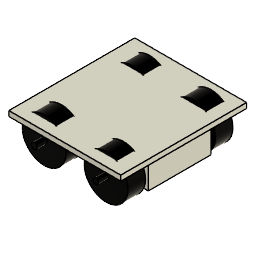
Bottom (Autodesk Fusion 360 design; units mm, degrees)
part number: 2026-06-28-07-39-42-404
Autodesk Fusion 360 part; units mm, degrees
sketch "Sketch1" plane through (0, 0, 0) normal (0, 0, 1) x (1, 0, 0)
  line L0 (0, 0) -> (72, 0)
  line L1 (72, 0) -> (72, 64)
  line L2 (72, 64) -> (0, 64)
  line L3 (0, 64) -> (0, 0)
  point P0 (9, 50)
  point P1 (63, 50)
  point P2 (9, 14)
  point P3 (63, 14)
  dimension "d1" = 72
  dimension "d2" = 64
  constraint horizontal L0
  constraint vertical L1
  constraint horizontal L2
  constraint vertical L3
  constraint coincident L0.start L3.end
  measures "d1" distance of L0.start L0.end
  measures "d2" distance of L0.start L2.end
extrude "Extrude1" add sketch "Sketch1" along normal blind 3 makes body 1
sketch "Sketch2" plane through (0, 0, 3) normal (0, 0, 1) x (-1, 0, 0)
  line L0 (0, -64) -> (0, 0)
  line L1 (0, 0) -> (-72, 0)
  line L2 (-72, 0) -> (-72, -64)
  line L3 (-72, -64) -> (0, -64)
  point P0 (-9, -50)
  point P1 (-9, -14)
  point P2 (-63, -49.8902)
  point P3 (-63, -14)
hole "Hole1" at (9, 50, 3) at (63, 49.8902, 3) at (63, 14, 3) at (9, 14, 3) direction (0, 0, -1) diameter 3.4 depth 3 tip angle 180 bodies 1
sketch "Sketch3" plane through (0, 0, 0) normal (0, 0, 1) x (1, 0, 0)
sketch "Sketch4" plane through (0, 0, 0) normal (1, 0, 0) x (0, 1, 0)
  line L0 (0, 11.5) -> (-48, 11.5)
  arc A0 (-48, 11.5) -> (-48, -11.5) centre (-48, 0) ccw
  line L1 (-48, -11.5) -> (0, -11.5)
  arc A1 (0, -11.5) -> (0, 11.5) centre (0, 0) ccw
  line L2 (0, 0) -> (-48, 0) construction
  dimension "d21" = 23
  constraint tangent L0 A0
  constraint tangent A0 L1
  constraint parallel L0 L1
  constraint tangent L1 A1
  constraint tangent L0 A1
  constraint horizontal L2
  constraint coincident A1.centre L2.start
  measures "d21" diameter of A0
ref_plane "WorkPlane1" through (0, -21.8422, 11.5) normal (0, -1, 0) x (1, 0, 0)
sketch "Sketch5" plane through (0, -21.8422, 11.5) normal (0, -1, 0) x (1, 0, 0)
  line L0 (0, 0) -> (-20, 0)
  line L1 (-20, 0) -> (-20, -2)
  line L2 (-20, -2) -> (0, -2)
  line L3 (0, -2) -> (0, 0)
  dimension "d23" = 2
  constraint horizontal L0
  constraint vertical L1
  constraint horizontal L2
  constraint vertical L3
  constraint coincident L0.start L3.end
  measures "d23" distance of L0.start L2.end
sketch "Sketch6" plane through (0, 0, 31.5) normal (0, 0, 1) x (-1, 0, 0)
sketch "Sketch7" plane through (0, 0, 31.5) normal (0, 0, 1) x (-1, 0, 0)
  line L0 (14.9741, -0.5329) -> (34.9741, -0.5329)
  line L1 (34.9741, -0.5329) -> (34.9741, 8.4671)
  line L2 (34.9741, 8.4671) -> (14.9741, 8.4671)
  line L3 (14.9741, 8.4671) -> (14.9741, -0.5329)
  dimension "d30" = 20
  dimension "d31" = 9
  constraint horizontal L0
  constraint vertical L1
  constraint horizontal L2
  constraint vertical L3
  measures "d30" distance of L0.start L0.end
  measures "d31" distance of L0.start L2.end
sketch "Sketch8" plane through (0, 0, 0) normal (1, 0, 0) x (0, 1, 0)
  circle A0 centre (-10, -10) radius 11
  dimension "d36" = 22
  measures "d36" diameter of A0
sketch "Sketch9" plane through (0, 0, 0) normal (1, 0, 0) x (0, 1, 0)
  circle A0 centre (-10, -10) radius 11
  dimension "d39" = 22
  measures "d39" diameter of A0
sketch "Sketch10" plane through (0, 0, 0) normal (1, 0, 0) x (0, 1, 0)
move_body "Move17" bodies 1 to x (1, 0, 0) y (0, 1, 0) z (0, 0, 1) at (-45, -55, 35)
sketch "Sketch11" plane through (0, 0, 0) normal (1, 0, 0) x (0, 1, 0)
move_body "Move18" bodies 1 to x (1, 0, 0) y (0, 1, 0) z (0, 0, 1) at (0, -70, 0)
move_body "Move19" bodies 1 to x (1, 0, 0) y (0, 1, 0) z (0, 0, 1) at (0, -5, 0)
sketch "Sketch12" plane through (0, 0, 0) normal (0, 0, 1) x (1, 0, 0)
  line L0 (-15, -55) -> (10, -55)
  line L1 (10, -55) -> (10, -27)
  line L2 (10, -27) -> (-15, -27)
  line L3 (-15, -27) -> (-15, -55)
  dimension "d50" = 25
  dimension "d51" = 28
  constraint horizontal L0
  constraint vertical L1
  constraint horizontal L2
  constraint vertical L3
  measures "d50" distance of L0.start L0.end
  measures "d51" distance of L0.start L2.end
move_body "Move21" bodies 1 to x (0, -1, 0) y (1, 0, 0) z (0, 0, 1) at (85, -95, 0)
sketch "Sketch13" plane through (0, 0, 35) normal (0, 0, -1) x (1, 0, 0)
  circle A0 centre (-31, 113) radius 1.7
  circle A1 centre (5, 59) radius 1.7
  circle A2 centre (4.8902, 113) radius 1.7
  circle A3 centre (-31, 59) radius 1.7
  line L0 (-45, 50) -> (19, 50)
  line L1 (19, 50) -> (19, 122)
  line L2 (19, 122) -> (-45, 122)
  line L3 (-45, 122) -> (-45, 50)
  circle A4 centre (0, 0) radius 1.5
  dimension "d56" = 3
  constraint coincident A4.centre origin
  measures "d56" diameter of A4
sketch "Sketch14" plane through (0, 0, 0) normal (0, 0, 1) x (1, 0, 0)
  circle A0 centre (35, -15) radius 20
  dimension "d59" = 40
  measures "d59" diameter of A0
sketch "Sketch15" plane through (0, 0, 0) normal (0, 1, 0) x (1, 0, 0)
  circle A0 centre (50, 25) radius 20
  dimension "d64" = 40
  measures "d64" diameter of A0
move_body "Move28" bodies 1 to x (1, 0, 0) y (0, 1, 0) z (0, 0, 1) at (5, 125, 20)
move_body "Move29" bodies 1 to x (1, 0, 0) y (0, 1, 0) z (0, 0, 1) at (-5, 1, 0)
move_body "Move30" bodies 1 to x (1, 0, 0) y (0, 1, 0) z (0, 0, 1) at (15, 0, 0)
sketch "Sketch16" plane through (0, 0, 58) normal (0, 0, 1) x (-1, 0, 0)
move_body "Move31" bodies 1 to x (1, 0, 0) y (0, 1, 0) z (0, 0, 1) at (70, 0, 0)
sketch "Sketch17" plane through (0, 0, 0) normal (0, 0, 1) x (1, 0, 0)
  line L0 (0, 0) -> (-39, 0)
  line L1 (-39, 0) -> (-39, 12)
  line L2 (-39, 12) -> (0, 12)
  line L3 (0, 12) -> (0, 0)
  line L4 (103.9674, 75.7753) -> (101.9674, 75.7753)
  line L5 (103.7737, 4.1752) -> (101.7737, 4.1752)
  line L6 (40, 76) -> (42, 76)
  line L7 (40, 4) -> (42, 4)
  line L8 (101.758, 57.9053) -> (42, 57.9053)
  line L9 (42, 57.9053) -> (42, 22)
  line L10 (42, 22) -> (101.758, 22)
  line L11 (101.758, 22) -> (101.758, 57.9053)
  dimension "d70" = 39
  dimension "d71" = 12
  constraint horizontal L0
  constraint vertical L1
  constraint horizontal L2
  constraint vertical L3
  constraint coincident L0.start L3.end
  constraint horizontal L6
  constraint horizontal L7
  constraint horizontal L8
  constraint vertical L9
  constraint horizontal L10
  constraint vertical L11
  measures "d70" distance of L0.start L0.end
  measures "d71" distance of L0.start L2.end
extrude "Extrude10" add sketch "Sketch17" along normal blind 15 separate body contours L8 L9 L10 L11 makes body 2
shell "Shell1" thickness 3 removed faces 1 at (61.9193, 45.9368, 15) on bodies 2
move_body "Move32" bodies 2 to x (1, 0, 0) y (0, 1, 0) z (0, 0, 1) at (0, 0, 40)
move_body "Move33" bodies 2 to x (1, 0, 0) y (0, 1, 0) z (0, 0, 1) at (0, -60, 0)
sketch "Sketch18" plane through (0, 0, 0) normal (0, 0, 1) x (1, 0, 0)
  line L0 (0, 0) -> (12, 0)
  line L1 (12, 0) -> (12, 39)
  line L2 (12, 39) -> (0, 39)
  line L3 (0, 39) -> (0, 0)
  dimension "d82" = 12
  dimension "d83" = 39
  constraint horizontal L0
  constraint vertical L1
  constraint horizontal L2
  constraint vertical L3
  constraint coincident L0.start L3.end
  measures "d82" distance of L0.start L0.end
  measures "d83" distance of L0.start L2.end
extrude "Extrude11" add sketch "Sketch18" along normal blind 12 separate body makes body 3
move_body "Move34" bodies 3 to x (0, 1, 0) y (-1, 0, 0) z (0, 0, 1) at (98.5, -17.5, 43)
sketch "Sketch19" plane through (0, 0, 0) normal (0, 0, 1) x (1, 0, 0)
  line L0 (0, 0) -> (12, 0)
  line L1 (12, 0) -> (12, 39)
  line L2 (12, 39) -> (0, 39)
  line L3 (0, 39) -> (0, 0)
  dimension "d86" = 12
  dimension "d87" = 39
  constraint horizontal L0
  constraint vertical L1
  constraint horizontal L2
  constraint vertical L3
  constraint coincident L0.start L3.end
  measures "d86" distance of L0.start L0.end
  measures "d87" distance of L0.start L2.end
extrude "Extrude12" add sketch "Sketch19" along normal blind 12 separate body makes body 4
move_body "Move35" bodies 4 to x (0, 1, 0) y (-1, 0, 0) z (0, 0, 1) at (98.319, -35.9909, 42)
move_body "Move36" bodies 4 to x (1, 0, 0) y (0, 1, 0) z (0, 0, 1) at (0, 0, 1)
move_body "Move37" bodies 4 to x (1, 0, 0) y (0, 1, 0) z (0, 0, 1) at (0, 1, 0)
move_body "Move38" bodies 1 to x (1, 0, 0) y (0, 1, 0) z (0, 0, 1) at (0, -60, 0)
sketch "Sketch20" plane through (0, -2.0947, 0) normal (0, 1, 0) x (-1, 0, 0)
  line L0 (-101.758, 40) -> (-42, 40)
  line L1 (-42, 40) -> (-42, 55)
  line L2 (-42, 55) -> (-101.758, 55)
  line L3 (-101.758, 55) -> (-101.758, 40)
  point P0 (-90, 47.5)
  point P1 (-54, 47.5)
hole "Hole6" at (54, -2.0947, 47.5) direction (0, -1, 0) diameter 3.4 depth 3 tip angle 180 bodies 2
sketch "Sketch21" plane through (0, -2.0947, 0) normal (0, 1, 0) x (-1, 0, 0)
  circle A0 centre (-54, 47.5) radius 1.7
  line L0 (-101.758, 40) -> (-42, 40)
  line L1 (-42, 40) -> (-42, 55)
  line L2 (-42, 55) -> (-101.758, 55)
  line L3 (-101.758, 55) -> (-101.758, 40)
  point P0 (-89.758, 47.5)
hole "Hole7" at (89.758, -2.0947, 47.5) direction (0, -1, 0) diameter 3 depth 3 tip angle 180 bodies 2
sketch "Sketch22" plane through (0, -38, 0) normal (0, -1, 0) x (1, 0, 0)
  line L0 (42, 40) -> (101.758, 40)
  line L1 (101.758, 40) -> (101.758, 55)
  line L2 (101.758, 55) -> (42, 55)
  line L3 (42, 55) -> (42, 40)
  line L4 (54, 55) -> (54, 47.5)
  line L5 (42, 47.5) -> (52.3, 47.5)
  point P0 (54, 47.5)
  dimension "d99" = 10.3
  constraint coincident L2 L4.start
  constraint midpoint L3 L5.start
  constraint perpendicular L4 L5
  constraint coincident P0 L4.end
  measures "d99" distance of L5.start L5.end
hole "Hole8" at (54, -38, 47.5) direction (0, 1, 0) diameter 3.4 depth 3 tip angle 180 bodies 2
sketch "Sketch23" plane through (0, -38, 0) normal (0, -1, 0) x (1, 0, 0)
  circle A0 centre (54, 47.5) radius 1.7
  line L0 (42, 40) -> (101.758, 40)
  line L1 (101.758, 40) -> (101.758, 55)
  line L2 (101.758, 55) -> (42, 55)
  line L3 (42, 55) -> (42, 40)
  point P0 (89.758, 47.5)
hole "Hole9" at (89.758, -38, 47.5) direction (0, 1, 0) diameter 3 depth 3 tip angle 180 bodies 2
move_body "Move39" bodies 1 to x (1, 0, 0) y (0, 1, 0) z (0, 0, 1) at (0, 70, 0)
move_body "Move40" bodies 1 to x (1, 0, 0) y (0, 1, 0) z (0, 0, 1) at (0, -70, 0)
sketch "Sketch24" plane through (0, 0, 0) normal (1, 0, 0) x (0, 1, 0)
  circle A0 centre (0, 25) radius 1.7
  dimension "d108" = 3.4
  measures "d108" diameter of A0
extrude "Extrude13" add sketch "Sketch24" along normal blind 72 separate body makes body 5
move_body "Move41" bodies 5 to x (0, 1, 0) y (-1, 0, 0) z (0, 0, 1) at (-1.7, -1.7, 0)
move_body "Move42" bodies 5 to x (1, 0, 0) y (0, 1, 0) z (0, 0, 1) at (55.8897, -54, 22.3906)
sketch "Sketch25" plane through (0, 0, 0) normal (1, 0, 0) x (0, 1, 0)
  circle A0 centre (0, 0) radius 1.5
  dimension "d111" = 3
  constraint coincident A0.centre origin
  measures "d111" diameter of A0
extrude "Extrude14" add sketch "Sketch25" along normal blind 72 separate body makes body 6
move_body "Move43" bodies 6 to x (0, -0.999993, 0.003779) y (0.999516, -0.000118, -0.031122) z (0.031122, 0.003777, 0.999508) at (0, -0.3423, 10.9947)
move_body "Move44" bodies 6 to x (1, 0, 0) y (0, 1, 0) z (0, 0, 1) at (89.6646, 16.4502, 36.5333)
sketch "Sketch26" plane through (0, 0, 0) normal (0, 1, 0) x (1, 0, 0)
  circle A0 centre (0, 0) radius 12.5
  dimension "d114" = 25
  constraint coincident A0.centre origin
  measures "d114" diameter of A0
extrude "Extrude15" add sketch "Sketch26" along normal blind 10 separate body makes body 7
move_body "Move45" bodies 7 to x (1, 0, 0) y (0, 1, 0) z (0, 0, 1) at (0, 0, 15)
hole "Hole10" at (0, 0, 15) direction (0, 1, 0) diameter 3.4 end through all bodies 7
move_body "Move46" bodies 7 to x (1, 0, 0) y (0, 1, 0) z (0, 0, 1) at (54.2242, -50, 32.3879)
sketch "Sketch27" plane through (0, 0, 0) normal (0, 1, 0) x (1, 0, 0)
  circle A0 centre (0, 0) radius 12.5
  dimension "d119" = 25
  constraint coincident A0.centre origin
  measures "d119" diameter of A0
extrude "Extrude16" add sketch "Sketch27" along normal blind 10 separate body makes body 8
hole "Hole11" at (0, 0, 0) direction (0, 1, 0) diameter 3.4 depth 10 tip angle 180 bodies 8
move_body "Move47" bodies 8 to x (1, 0, 0) y (0, 1, 0) z (0, 0, 1) at (54.5668, 0, 46.9757)
sketch "Sketch28" plane through (0, 0, 0) normal (0, 1, 0) x (1, 0, 0)
  circle A0 centre (0, 0) radius 12.5
  dimension "d125" = 25
  constraint coincident A0.centre origin
  measures "d125" diameter of A0
extrude "Extrude17" add sketch "Sketch28" along normal blind 10 separate body makes body 9
move_body "Move48" bodies 9 to x (1, 0, 0) y (0, 1, 0) z (0, 0, 1) at (-5.0166, 50, 19.3606)
hole "Hole12" at (-5.0166, 60, 19.3606) direction (0, -1, 0) diameter 3 end through all bodies 9
move_body "Move49" bodies 9 to x (1, 0, 0) y (0, 1, 0) z (0, 0, 1) at (94.6576, -50, 28.2499)
sketch "Sketch29" plane through (0, 0, 0) normal (0, 1, 0) x (1, 0, 0)
  circle A0 centre (0, 0) radius 12.5
  dimension "d130" = 25
  constraint coincident A0.centre origin
  measures "d130" diameter of A0
extrude "Extrude18" add sketch "Sketch29" along normal blind 10 separate body makes body 10
hole "Hole13" at (0, 0, 0) direction (0, 1, 0) diameter 3 end through all bodies 10
move_body "Move50" bodies 10 to x (1, 0, 0) y (0, 1, 0) z (0, 0, 1) at (89.618, -50, 46.9293)
named bodies: "N20 motor"
